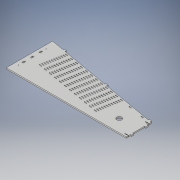
# Autodesk Inventor part: pinball-case-left-wall
Saved by Autodesk Inventor 2017 (Build 210142000, 142)
## iProperties
Created: 2017-02-27
Part Number: pinball-case-left-wall
Material: Generic
Document SubType Name: Modeling
Designer: John
Density: 1 g/cm^3
Appearance: Default
Author: John
Autodesk Inventor part; units mm, degrees
ref_plane "YZ Plane" through (0, 0, 0) normal (1, 0, 0) x (0, 1, 0)
ref_plane "XZ Plane" through (0, 0, 0) normal (0, 1, 0) x (-1, 0, 0)
ref_plane "XY Plane" through (0, 0, 0) normal (0, 0, 1) x (1, 0, 0)
sketch "Sketch1" plane through (0, 0, 0) normal (0, 1, 0) x (-1, 0, 0)
  line L0 (0, 0) -> (-590, 0)
  line L1 (-590, 0) -> (-590, -120.9671)
  line L2 (-590, -120.9671) -> (0, -120.9671)
  line L3 (0, -120.9671) -> (0, 0)
  line L4 (0, -120.9671) -> (0, -225)
  line L5 (0, -225) -> (-590, -120.9671)
  dimension "d0" = 590
  dimension "d50" = 225
  dimension "d51" = 10
  constraints: 12 end point, 2 parallel, 1 horizontal, 1 perpendicular, 1 vertical
  measures "d0" distance of L2.end L1.end
  measures "d50" distance of L0.start L4.end
  measures "d51" angle of L2 L5
extrude "Extrusion1" add sketch "Sketch1" along normal blind 6
sketch "Sketch2" plane through (0, 6, 0) normal (0, 1, 0) x (1, 0, 0)
  line L0 (62.143, 214.0425) -> (73.9607, 211.9587)
  line L1 (73.9607, 211.9587) -> (75.0026, 217.8676)
  line L2 (75.0026, 217.8676) -> (63.1849, 219.9514)
  line L3 (63.1849, 219.9514) -> (62.143, 214.0425)
  line L4 (0, 225) -> (62.143, 214.0425) construction
  line L5 (590, 120.9671) -> (578.1823, 123.0509) construction
  line L6 (590, 120.9671) -> (0, 225) construction
  line L7 (578.1823, 123.0509) -> (566.3646, 125.1346)
  line L8 (566.3646, 125.1346) -> (567.4065, 131.0435)
  line L9 (567.4065, 131.0435) -> (579.2242, 128.9597)
  line L10 (579.2242, 128.9597) -> (578.1823, 123.0509)
  line L11 (320.1627, 168.5467) -> (308.345, 170.6305)
  line L12 (308.345, 170.6305) -> (309.3869, 176.5393)
  line L13 (309.3869, 176.5393) -> (321.2046, 174.4555)
  line L14 (321.2046, 174.4555) -> (320.1627, 168.5467)
  point P0 (0, 0)
  dimension "d5" = 6
  dimension "d7" = 12
  dimension "d9" = 12
  dimension "d10" = 12
  dimension "d11" = 6
  dimension "d14" = 500
  dimension "d15" = 12
  dimension "d16" = 6
  dimension "d17" = 250
  constraints: 28 end point, 6 parallel, 3 perpendicular, 3 point on line, 1 collinear
  measures "d5" distance of L1.end L0.end
  measures "d7" distance between parallel lines of L1 L3
  measures "d9" distance of L5.start L5.end
  measures "d10" distance of L5.end L7.end
  measures "d11" distance of L7.end L8.end
  measures "d14" distance between parallel lines of L8 L1
  measures "d15" distance of L11.start L11.end
  measures "d16" distance of L11.end L12.end
  measures "d17" distance between parallel lines of L14 L8
extrude "Extrusion2" add sketch "Sketch2" against normal blind 6
sketch "Sketch3" plane through (0, 6, 0) normal (0, 1, 0) x (1, 0, 0)
  line L0 (590, 0) -> (590, 120.9671) projected
  line L1 (590, 126) -> (584, 126)
  line L2 (584, 126) -> (584, 101)
  line L3 (584, 101) -> (590, 101)
  line L4 (590, 101) -> (590, 126)
  line L5 (590, 0) -> (584, 0)
  line L6 (584, 0) -> (584, 20)
  line L7 (584, 20) -> (590, 20)
  line L8 (590, 20) -> (590, 0)
  line L9 (590, 89) -> (584, 89)
  line L10 (584, 89) -> (584, 32)
  line L11 (584, 32) -> (590, 32)
  line L12 (590, 32) -> (590, 89)
  point P0 (0, 0)
  dimension "d18" = 6
  dimension "d20" = 6
  dimension "d21" = 20
  dimension "d22" = 12
  dimension "d23" = 12
  dimension "d27" = 57
  dimension "d36" = 25
  constraints: 24 end point, 6 parallel, 3 horizontal, 3 perpendicular, 1 point on line
  measures "d18" distance of L3.end L2.end
  measures "d20" distance of L6.end L7.end
  measures "d21" distance of L5.end L6.end
  measures "d22" distance between parallel lines of L3 L9
  measures "d23" distance between parallel lines of L7 L11
  measures "d27" distance of L9.end L10.end
  measures "d36" distance of L1.end L2.end
extrude "Extrusion3" cut sketch "Sketch3" along normal through all both and the other way through all
sketch "Sketch4" plane through (0, 6, 0) normal (0, 1, 0) x (1, 0, 0)
  line L0 (584, 0) -> (584, 20) projected
  line L1 (584, 12) -> (576, 12)
  line L2 (567, 12) -> (567, 9.5)
  line L3 (567, 9.5) -> (573.7, 9.5)
  line L4 (584, 9.5) -> (584, 12)
  line L5 (0, 0) -> (584, 0) construction
  line L6 (573.7, 13.45) -> (576, 13.45)
  line L7 (576, 13.45) -> (576, 12)
  line L8 (576, 8.05) -> (573.7, 8.05)
  line L9 (573.7, 8.05) -> (573.7, 9.5)
  line L10 (576, 12) -> (576, 9.5) construction
  line L11 (576, 9.5) -> (576, 8.05)
  line L12 (573.7, 12) -> (573.7, 13.45)
  line L13 (573.7, 9.5) -> (573.7, 12) construction
  line L14 (576, 12) -> (573.7, 12) construction
  line L15 (573.7, 12) -> (567, 12)
  line L16 (576, 9.5) -> (584, 9.5)
  line L17 (573.7, 9.5) -> (576, 9.5) construction
  line L18 (584, 111.5) -> (576, 111.5)
  line L19 (567, 111.5) -> (567, 109)
  line L20 (567, 109) -> (573.7, 109)
  line L21 (584, 109) -> (584, 111.5)
  line L22 (573.7, 112.95) -> (576, 112.95)
  line L23 (576, 112.95) -> (576, 111.5)
  line L24 (576, 107.55) -> (573.7, 107.55)
  line L25 (573.7, 107.55) -> (573.7, 109)
  line L26 (576, 111.5) -> (576, 109) construction
  line L27 (576, 109) -> (576, 107.55)
  line L28 (573.7, 111.5) -> (573.7, 112.95)
  line L29 (573.7, 109) -> (573.7, 111.5) construction
  line L30 (576, 111.5) -> (573.7, 111.5) construction
  line L31 (573.7, 111.5) -> (567, 111.5)
  line L32 (576, 109) -> (584, 109)
  line L33 (573.7, 109) -> (576, 109) construction
  line L34 (590, 101) -> (584, 101) construction
  line L35 (584, 20) -> (590, 20) construction
  line L36 (14.1705, 156) -> (20.1705, 156)
  line L37 (20.1705, 156) -> (20.1705, 144)
  line L38 (20.1705, 144) -> (14.1705, 144)
  line L39 (14.1705, 144) -> (14.1705, 156)
  line L40 (15, 114) -> (21, 114)
  line L41 (21, 114) -> (21, 102)
  line L42 (21, 102) -> (15, 102)
  line L43 (15, 102) -> (15, 114)
  line L44 (15, 72) -> (21, 72)
  line L45 (21, 72) -> (21, 60)
  line L46 (21, 60) -> (15, 60)
  line L47 (15, 60) -> (15, 72)
  line L48 (0, 225) -> (0, 0) projected
  circle A0 centre (17.1705, 176) radius 1.25
  circle A1 centre (18, 40) radius 1.25
  line L49 (18, 60) -> (18, 40) construction
  point P0 (584, 122.025)
  dimension "d37" = 17
  dimension "d38" = 2.5
  dimension "d58" = 2.3
  dimension "d59" = 5.4
  dimension "d60" = 8
  dimension "d66" = 17
  dimension "d67" = 2.5
  dimension "d68" = 2.3
  dimension "d69" = 5.4
  dimension "d70" = 8
  dimension "d71" = 8
  dimension "d72" = 6
  dimension "d73" = 12
  dimension "d77" = 30
  dimension "d78" = 30
  dimension "d79" = 60
  dimension "d80" = 15
  dimension "d81" = 2.5
  dimension "d82" = 2.5
  dimension "d83" = 20
  dimension "d84" = 20
  constraints: 90 end point, 46 parallel, 15 perpendicular, 11 horizontal, 5 equal length, 5 point on line, 2 centre point, 1 midpoint, 1 vertical
  measures "d37" distance of L4.start L2.end
  measures "d38" distance of L2.end L2.start
  measures "d58" distance of L8.start L8.end
  measures "d59" distance of L6.end L8.start
  measures "d60" distance between parallel lines of L0 L7
  measures "d66" distance of L21.start L19.end
  measures "d67" distance of L19.end L31.end
  measures "d68" distance of L24.start L24.end
  measures "d69" distance of L22.end L24.start
  measures "d70" distance between parallel lines of L34 L32
  measures "d71" distance between parallel lines of L1 L35
  measures "d72" distance of L37.end L38.end
  measures "d73" distance of L36.end L37.end
  measures "d77" distance between parallel lines of L38 L40
  measures "d78" distance between parallel lines of L44 L42
  measures "d79" distance between parallel lines of L46 L5
  measures "d80" distance between parallel lines of L48 L47
  measures "d81" diameter of A0
  measures "d82" diameter of A1
  measures "d83" distance from line of L49.end L46
  measures "d84" distance from line of L36 A0.centre
extrude "Extrusion4" cut sketch "Sketch4" along normal through all both and the other way through all
sketch "Sketch5" plane through (0, 6, 0) normal (0, 1, 0) x (1, 0, 0)
  circle A0 centre (490, 60) radius 12
  line L0 (0, 0) -> (584, 0) projected
  line L1 (590, 89) -> (590, 101) projected
  dimension "d45" = 24
  dimension "d46" = 60
  dimension "d47" = 100
  constraints: 1 centre point
  measures "d45" diameter of A0
  measures "d46" distance from line of L0 A0.centre
  measures "d47" distance from line of L1 A0.centre
extrude "Extrusion5" cut sketch "Sketch5" against normal through all
sketch "Sketch6" plane through (0, 6, 0) normal (0, 1, 0) x (1, 0, 0)
  line L0 (533.8089, 124.7825) -> (545.6266, 122.6988)
  line L1 (545.6266, 122.6988) -> (545.1056, 119.7443)
  line L2 (545.1056, 119.7443) -> (533.2879, 121.8281)
  line L3 (533.2879, 121.8281) -> (533.8089, 124.7825)
  line L4 (474.7204, 135.2014) -> (462.9027, 137.2852)
  line L5 (462.9027, 137.2852) -> (462.3818, 134.3308)
  line L6 (462.3818, 134.3308) -> (474.1995, 132.247)
  line L7 (474.1995, 132.247) -> (474.7204, 135.2014)
  line L8 (566.3646, 125.1346) -> (320.1627, 168.5467) projected
  point P0 (0, 0)
  dimension "d85" = 12
  dimension "d86" = 3
  dimension "d87" = 12
  dimension "d88" = 60
  dimension "d89" = 20
  dimension "d92" = 6
  constraints: 16 end point, 5 parallel, 2 perpendicular, 2 point on line, 1 collinear
  measures "d85" distance of L1.end L2.end
  measures "d86" distance of L0.end L1.end
  measures "d87" distance of L6.end L5.end
  measures "d88" distance between parallel lines of L7 L3
  measures "d89" distance from line of L1 L8.start
  measures "d92" distance between parallel lines of L0 L8
extrude "Extrusion6" cut sketch "Sketch6" against normal through all
sketch "Sketch7" plane through (0, 6, 0) normal (0, 1, 0) x (1, 0, 0)
  line L0 (422.9895, 141.2767) -> (411.1718, 143.3605)
  line L1 (411.1718, 143.3605) -> (411.6927, 146.3149)
  line L2 (411.6927, 146.3149) -> (423.5104, 144.2311)
  line L3 (423.5104, 144.2311) -> (422.9895, 141.2767)
  line L4 (462.9027, 137.2852) -> (474.7204, 135.2014) projected
  line L5 (566.3646, 125.1346) -> (320.1627, 168.5467) projected
  line L6 (421.253, 131.4286) -> (409.4353, 133.5124)
  line L7 (409.4353, 133.5124) -> (409.9562, 136.4668)
  line L8 (409.9562, 136.4668) -> (421.7739, 134.3831)
  line L9 (421.7739, 134.3831) -> (421.253, 131.4286)
  line L10 (419.5165, 121.5806) -> (407.6988, 123.6643)
  line L11 (407.6988, 123.6643) -> (408.2198, 126.6188)
  line L12 (408.2198, 126.6188) -> (420.0374, 124.535)
  line L13 (420.0374, 124.535) -> (419.5165, 121.5806)
  line L14 (417.78, 111.7325) -> (405.9623, 113.8163)
  line L15 (405.9623, 113.8163) -> (406.4833, 116.7707)
  line L16 (406.4833, 116.7707) -> (418.301, 114.6869)
  line L17 (418.301, 114.6869) -> (417.78, 111.7325)
  line L18 (416.0435, 101.8844) -> (404.2258, 103.9682)
  line L19 (404.2258, 103.9682) -> (404.7468, 106.9226)
  line L20 (404.7468, 106.9226) -> (416.5645, 104.8388)
  line L21 (416.5645, 104.8388) -> (416.0435, 101.8844)
  line L22 (414.3071, 92.0363) -> (402.4894, 94.1201)
  line L23 (402.4894, 94.1201) -> (403.0103, 97.0745)
  line L24 (403.0103, 97.0745) -> (414.828, 94.9907)
  line L25 (414.828, 94.9907) -> (414.3071, 92.0363)
  line L26 (412.5706, 82.1882) -> (400.7529, 84.272)
  line L27 (400.7529, 84.272) -> (401.2738, 87.2264)
  line L28 (401.2738, 87.2264) -> (413.0915, 85.1427)
  line L29 (413.0915, 85.1427) -> (412.5706, 82.1882)
  line L30 (410.8341, 72.3402) -> (399.0164, 74.4239)
  line L31 (399.0164, 74.4239) -> (399.5373, 77.3784)
  line L32 (399.5373, 77.3784) -> (411.355, 75.2946)
  line L33 (411.355, 75.2946) -> (410.8341, 72.3402)
  line L34 (393.4452, 146.4862) -> (381.6275, 148.5699)
  line L35 (381.6275, 148.5699) -> (382.1485, 151.5244)
  line L36 (382.1485, 151.5244) -> (393.9662, 149.4406)
  line L37 (393.9662, 149.4406) -> (393.4452, 146.4862)
  line L38 (391.7087, 136.6381) -> (379.8911, 138.7219)
  line L39 (379.8911, 138.7219) -> (380.412, 141.6763)
  line L40 (380.412, 141.6763) -> (392.2297, 139.5925)
  line L41 (392.2297, 139.5925) -> (391.7087, 136.6381)
  line L42 (389.9723, 126.79) -> (378.1546, 128.8738)
  line L43 (378.1546, 128.8738) -> (378.6755, 131.8282)
  line L44 (378.6755, 131.8282) -> (390.4932, 129.7444)
  line L45 (390.4932, 129.7444) -> (389.9723, 126.79)
  line L46 (388.2358, 116.9419) -> (376.4181, 119.0257)
  line L47 (376.4181, 119.0257) -> (376.939, 121.9801)
  line L48 (376.939, 121.9801) -> (388.7567, 119.8963)
  line L49 (388.7567, 119.8963) -> (388.2358, 116.9419)
  line L50 (386.4993, 107.0938) -> (374.6816, 109.1776)
  line L51 (374.6816, 109.1776) -> (375.2026, 112.132)
  line L52 (375.2026, 112.132) -> (387.0202, 110.0483)
  line L53 (387.0202, 110.0483) -> (386.4993, 107.0938)
  line L54 (384.7628, 97.2458) -> (372.9451, 99.3295)
  line L55 (372.9451, 99.3295) -> (373.4661, 102.284)
  line L56 (373.4661, 102.284) -> (385.2838, 100.2002)
  line L57 (385.2838, 100.2002) -> (384.7628, 97.2458)
  line L58 (383.0263, 87.3977) -> (371.2086, 89.4815)
  line L59 (371.2086, 89.4815) -> (371.7296, 92.4359)
  line L60 (371.7296, 92.4359) -> (383.5473, 90.3521)
  line L61 (383.5473, 90.3521) -> (383.0263, 87.3977)
  line L62 (381.2899, 77.5496) -> (369.4722, 79.6334)
  line L63 (369.4722, 79.6334) -> (369.9931, 82.5878)
  line L64 (369.9931, 82.5878) -> (381.8108, 80.504)
  line L65 (381.8108, 80.504) -> (381.2899, 77.5496)
  line L66 (363.901, 151.6956) -> (352.0833, 153.7794)
  line L67 (352.0833, 153.7794) -> (352.6043, 156.7338)
  line L68 (352.6043, 156.7338) -> (364.4219, 154.65)
  line L69 (364.4219, 154.65) -> (363.901, 151.6956)
  line L70 (362.1645, 141.8475) -> (350.3468, 143.9313)
  line L71 (350.3468, 143.9313) -> (350.8678, 146.8857)
  line L72 (350.8678, 146.8857) -> (362.6855, 144.8019)
  line L73 (362.6855, 144.8019) -> (362.1645, 141.8475)
  line L74 (360.428, 131.9994) -> (348.6103, 134.0832)
  line L75 (348.6103, 134.0832) -> (349.1313, 137.0376)
  line L76 (349.1313, 137.0376) -> (360.949, 134.9539)
  line L77 (360.949, 134.9539) -> (360.428, 131.9994)
  line L78 (358.6916, 122.1514) -> (346.8739, 124.2351)
  line L79 (346.8739, 124.2351) -> (347.3948, 127.1896)
  line L80 (347.3948, 127.1896) -> (359.2125, 125.1058)
  line L81 (359.2125, 125.1058) -> (358.6916, 122.1514)
  line L82 (356.9551, 112.3033) -> (345.1374, 114.3871)
  line L83 (345.1374, 114.3871) -> (345.6583, 117.3415)
  line L84 (345.6583, 117.3415) -> (357.476, 115.2577)
  line L85 (357.476, 115.2577) -> (356.9551, 112.3033)
  line L86 (355.2186, 102.4552) -> (343.4009, 104.539)
  line L87 (343.4009, 104.539) -> (343.9218, 107.4934)
  line L88 (343.9218, 107.4934) -> (355.7395, 105.4096)
  line L89 (355.7395, 105.4096) -> (355.2186, 102.4552)
  line L90 (353.4821, 92.6071) -> (341.6644, 94.6909)
  line L91 (341.6644, 94.6909) -> (342.1854, 97.6453)
  line L92 (342.1854, 97.6453) -> (354.0031, 95.5616)
  line L93 (354.0031, 95.5616) -> (353.4821, 92.6071)
  line L94 (351.7456, 82.7591) -> (339.9279, 84.8428)
  line L95 (339.9279, 84.8428) -> (340.4489, 87.7973)
  line L96 (340.4489, 87.7973) -> (352.2666, 85.7135)
  line L97 (352.2666, 85.7135) -> (351.7456, 82.7591)
  line L98 (334.3568, 156.905) -> (322.5391, 158.9888)
  line L99 (322.5391, 158.9888) -> (323.06, 161.9432)
  line L100 (323.06, 161.9432) -> (334.8777, 159.8595)
  line L101 (334.8777, 159.8595) -> (334.3568, 156.905)
  line L102 (332.6203, 147.057) -> (320.8026, 149.1407)
  line L103 (320.8026, 149.1407) -> (321.3235, 152.0952)
  line L104 (321.3235, 152.0952) -> (333.1412, 150.0114)
  line L105 (333.1412, 150.0114) -> (332.6203, 147.057)
  line L106 (330.8838, 137.2089) -> (319.0661, 139.2927)
  line L107 (319.0661, 139.2927) -> (319.5871, 142.2471)
  line L108 (319.5871, 142.2471) -> (331.4047, 140.1633)
  line L109 (331.4047, 140.1633) -> (330.8838, 137.2089)
  line L110 (329.1473, 127.3608) -> (317.3296, 129.4446)
  line L111 (317.3296, 129.4446) -> (317.8506, 132.399)
  line L112 (317.8506, 132.399) -> (329.6683, 130.3152)
  line L113 (329.6683, 130.3152) -> (329.1473, 127.3608)
  line L114 (327.4108, 117.5127) -> (315.5931, 119.5965)
  line L115 (315.5931, 119.5965) -> (316.1141, 122.5509)
  line L116 (316.1141, 122.5509) -> (327.9318, 120.4672)
  line L117 (327.9318, 120.4672) -> (327.4108, 117.5127)
  line L118 (325.6744, 107.6647) -> (313.8567, 109.7484)
  line L119 (313.8567, 109.7484) -> (314.3776, 112.7029)
  line L120 (314.3776, 112.7029) -> (326.1953, 110.6191)
  line L121 (326.1953, 110.6191) -> (325.6744, 107.6647)
  line L122 (323.9379, 97.8166) -> (312.1202, 99.9004)
  line L123 (312.1202, 99.9004) -> (312.6411, 102.8548)
  line L124 (312.6411, 102.8548) -> (324.4588, 100.771)
  line L125 (324.4588, 100.771) -> (323.9379, 97.8166)
  line L126 (322.2014, 87.9685) -> (310.3837, 90.0523)
  line L127 (310.3837, 90.0523) -> (310.9046, 93.0067)
  line L128 (310.9046, 93.0067) -> (322.7223, 90.9229)
  line L129 (322.7223, 90.9229) -> (322.2014, 87.9685)
  line L130 (304.8125, 162.1145) -> (292.9948, 164.1983)
  line L131 (292.9948, 164.1983) -> (293.5158, 167.1527)
  line L132 (293.5158, 167.1527) -> (305.3335, 165.0689)
  line L133 (305.3335, 165.0689) -> (304.8125, 162.1145)
  line L134 (303.0761, 152.2664) -> (291.2584, 154.3502)
  line L135 (291.2584, 154.3502) -> (291.7793, 157.3046)
  line L136 (291.7793, 157.3046) -> (303.597, 155.2208)
  line L137 (303.597, 155.2208) -> (303.0761, 152.2664)
  line L138 (301.3396, 142.4183) -> (289.5219, 144.5021)
  line L139 (289.5219, 144.5021) -> (290.0428, 147.4565)
  line L140 (290.0428, 147.4565) -> (301.8605, 145.3728)
  line L141 (301.8605, 145.3728) -> (301.3396, 142.4183)
  line L142 (299.6031, 132.5703) -> (287.7854, 134.654)
  line L143 (287.7854, 134.654) -> (288.3063, 137.6085)
  line L144 (288.3063, 137.6085) -> (300.124, 135.5247)
  line L145 (300.124, 135.5247) -> (299.6031, 132.5703)
  line L146 (297.8666, 122.7222) -> (286.0489, 124.806)
  line L147 (286.0489, 124.806) -> (286.5699, 127.7604)
  line L148 (286.5699, 127.7604) -> (298.3876, 125.6766)
  line L149 (298.3876, 125.6766) -> (297.8666, 122.7222)
  line L150 (296.1301, 112.8741) -> (284.3124, 114.9579)
  line L151 (284.3124, 114.9579) -> (284.8334, 117.9123)
  line L152 (284.8334, 117.9123) -> (296.6511, 115.8285)
  line L153 (296.6511, 115.8285) -> (296.1301, 112.8741)
  line L154 (294.3936, 103.026) -> (282.5759, 105.1098)
  line L155 (282.5759, 105.1098) -> (283.0969, 108.0642)
  line L156 (283.0969, 108.0642) -> (294.9146, 105.9804)
  line L157 (294.9146, 105.9804) -> (294.3936, 103.026)
  line L158 (292.6572, 93.1779) -> (280.8395, 95.2617)
  line L159 (280.8395, 95.2617) -> (281.3604, 98.2161)
  line L160 (281.3604, 98.2161) -> (293.1781, 96.1324)
  line L161 (293.1781, 96.1324) -> (292.6572, 93.1779)
  line L162 (275.2683, 167.3239) -> (263.4506, 169.4077)
  line L163 (263.4506, 169.4077) -> (263.9716, 172.3621)
  line L164 (263.9716, 172.3621) -> (275.7892, 170.2784)
  line L165 (275.7892, 170.2784) -> (275.2683, 167.3239)
  line L166 (273.5318, 157.4759) -> (261.7141, 159.5596)
  line L167 (261.7141, 159.5596) -> (262.2351, 162.5141)
  line L168 (262.2351, 162.5141) -> (274.0528, 160.4303)
  line L169 (274.0528, 160.4303) -> (273.5318, 157.4759)
  line L170 (271.7953, 147.6278) -> (259.9776, 149.7116)
  line L171 (259.9776, 149.7116) -> (260.4986, 152.666)
  line L172 (260.4986, 152.666) -> (272.3163, 150.5822)
  line L173 (272.3163, 150.5822) -> (271.7953, 147.6278)
  line L174 (270.0589, 137.7797) -> (258.2412, 139.8635)
  line L175 (258.2412, 139.8635) -> (258.7621, 142.8179)
  line L176 (258.7621, 142.8179) -> (270.5798, 140.7341)
  line L177 (270.5798, 140.7341) -> (270.0589, 137.7797)
  line L178 (268.3224, 127.9316) -> (256.5047, 130.0154)
  line L179 (256.5047, 130.0154) -> (257.0256, 132.9698)
  line L180 (257.0256, 132.9698) -> (268.8433, 130.886)
  line L181 (268.8433, 130.886) -> (268.3224, 127.9316)
  line L182 (266.5859, 118.0835) -> (254.7682, 120.1673)
  line L183 (254.7682, 120.1673) -> (255.2891, 123.1217)
  line L184 (255.2891, 123.1217) -> (267.1068, 121.038)
  line L185 (267.1068, 121.038) -> (266.5859, 118.0835)
  line L186 (264.8494, 108.2355) -> (253.0317, 110.3192)
  line L187 (253.0317, 110.3192) -> (253.5527, 113.2737)
  line L188 (253.5527, 113.2737) -> (265.3704, 111.1899)
  line L189 (265.3704, 111.1899) -> (264.8494, 108.2355)
  line L190 (263.1129, 98.3874) -> (251.2952, 100.4712)
  line L191 (251.2952, 100.4712) -> (251.8162, 103.4256)
  line L192 (251.8162, 103.4256) -> (263.6339, 101.3418)
  line L193 (263.6339, 101.3418) -> (263.1129, 98.3874)
  line L194 (245.7241, 172.5334) -> (233.9064, 174.6172)
  line L195 (233.9064, 174.6172) -> (234.4273, 177.5716)
  line L196 (234.4273, 177.5716) -> (246.245, 175.4878)
  line L197 (246.245, 175.4878) -> (245.7241, 172.5334)
  line L198 (243.9876, 162.6853) -> (232.1699, 164.7691)
  line L199 (232.1699, 164.7691) -> (232.6908, 167.7235)
  line L200 (232.6908, 167.7235) -> (244.5085, 165.6397)
  line L201 (244.5085, 165.6397) -> (243.9876, 162.6853)
  line L202 (242.2511, 152.8372) -> (230.4334, 154.921)
  line L203 (230.4334, 154.921) -> (230.9544, 157.8754)
  line L204 (230.9544, 157.8754) -> (242.772, 155.7916)
  line L205 (242.772, 155.7916) -> (242.2511, 152.8372)
  line L206 (240.5146, 142.9891) -> (228.6969, 145.0729)
  line L207 (228.6969, 145.0729) -> (229.2179, 148.0273)
  line L208 (229.2179, 148.0273) -> (241.0356, 145.9436)
  line L209 (241.0356, 145.9436) -> (240.5146, 142.9891)
  line L210 (238.7781, 133.1411) -> (226.9604, 135.2248)
  line L211 (226.9604, 135.2248) -> (227.4814, 138.1793)
  line L212 (227.4814, 138.1793) -> (239.2991, 136.0955)
  line L213 (239.2991, 136.0955) -> (238.7781, 133.1411)
  line L214 (237.0417, 123.293) -> (225.224, 125.3768)
  line L215 (225.224, 125.3768) -> (225.7449, 128.3312)
  line L216 (225.7449, 128.3312) -> (237.5626, 126.2474)
  line L217 (237.5626, 126.2474) -> (237.0417, 123.293)
  line L218 (235.3052, 113.4449) -> (223.4875, 115.5287)
  line L219 (223.4875, 115.5287) -> (224.0084, 118.4831)
  line L220 (224.0084, 118.4831) -> (235.8261, 116.3993)
  line L221 (235.8261, 116.3993) -> (235.3052, 113.4449)
  line L222 (233.5687, 103.5968) -> (221.751, 105.6806)
  line L223 (221.751, 105.6806) -> (222.2719, 108.635)
  line L224 (222.2719, 108.635) -> (234.0896, 106.5513)
  line L225 (234.0896, 106.5513) -> (233.5687, 103.5968)
  line L226 (216.1798, 177.7428) -> (204.3621, 179.8266)
  line L227 (204.3621, 179.8266) -> (204.8831, 182.781)
  line L228 (204.8831, 182.781) -> (216.7008, 180.6972)
  line L229 (216.7008, 180.6972) -> (216.1798, 177.7428)
  line L230 (214.4434, 167.8947) -> (202.6257, 169.9785)
  line L231 (202.6257, 169.9785) -> (203.1466, 172.9329)
  line L232 (203.1466, 172.9329) -> (214.9643, 170.8492)
  line L233 (214.9643, 170.8492) -> (214.4434, 167.8947)
  line L234 (212.7069, 158.0467) -> (200.8892, 160.1304)
  line L235 (200.8892, 160.1304) -> (201.4101, 163.0849)
  line L236 (201.4101, 163.0849) -> (213.2278, 161.0011)
  line L237 (213.2278, 161.0011) -> (212.7069, 158.0467)
  line L238 (210.9704, 148.1986) -> (199.1527, 150.2824)
  line L239 (199.1527, 150.2824) -> (199.6736, 153.2368)
  line L240 (199.6736, 153.2368) -> (211.4913, 151.153)
  line L241 (211.4913, 151.153) -> (210.9704, 148.1986)
  line L242 (209.2339, 138.3505) -> (197.4162, 140.4343)
  line L243 (197.4162, 140.4343) -> (197.9372, 143.3887)
  line L244 (197.9372, 143.3887) -> (209.7549, 141.3049)
  line L245 (209.7549, 141.3049) -> (209.2339, 138.3505)
  line L246 (207.4974, 128.5024) -> (195.6797, 130.5862)
  line L247 (195.6797, 130.5862) -> (196.2007, 133.5406)
  line L248 (196.2007, 133.5406) -> (208.0184, 131.4569)
  line L249 (208.0184, 131.4569) -> (207.4974, 128.5024)
  line L250 (205.7609, 118.6544) -> (193.9433, 120.7381)
  line L251 (193.9433, 120.7381) -> (194.4642, 123.6926)
  line L252 (194.4642, 123.6926) -> (206.2819, 121.6088)
  line L253 (206.2819, 121.6088) -> (205.7609, 118.6544)
  line L254 (204.0245, 108.8063) -> (192.2068, 110.8901)
  line L255 (192.2068, 110.8901) -> (192.7277, 113.8445)
  line L256 (192.7277, 113.8445) -> (204.5454, 111.7607)
  line L257 (204.5454, 111.7607) -> (204.0245, 108.8063)
  line L258 (462.3818, 134.3308) -> (462.9027, 137.2852) projected
  line L259 (409.0976, 62.4921) -> (397.2799, 64.5759)
  line L260 (397.2799, 64.5759) -> (397.8009, 67.5303)
  line L261 (397.8009, 67.5303) -> (409.6186, 65.4465)
  line L262 (409.6186, 65.4465) -> (409.0976, 62.4921)
  line L263 (379.5534, 67.7015) -> (367.7357, 69.7853)
  line L264 (367.7357, 69.7853) -> (368.2566, 72.7397)
  line L265 (368.2566, 72.7397) -> (380.0743, 70.656)
  line L266 (380.0743, 70.656) -> (379.5534, 67.7015)
  line L267 (350.0091, 72.911) -> (338.1915, 74.9948)
  line L268 (338.1915, 74.9948) -> (338.7124, 77.9492)
  line L269 (338.7124, 77.9492) -> (350.5301, 75.8654)
  line L270 (350.5301, 75.8654) -> (350.0091, 72.911)
  line L271 (320.4649, 78.1204) -> (308.6472, 80.2042)
  line L272 (308.6472, 80.2042) -> (309.1682, 83.1586)
  line L273 (309.1682, 83.1586) -> (320.9859, 81.0748)
  line L274 (320.9859, 81.0748) -> (320.4649, 78.1204)
  line L275 (290.9207, 83.3299) -> (279.103, 85.4136)
  line L276 (279.103, 85.4136) -> (279.6239, 88.3681)
  line L277 (279.6239, 88.3681) -> (291.4416, 86.2843)
  line L278 (291.4416, 86.2843) -> (290.9207, 83.3299)
  line L279 (261.3764, 88.5393) -> (249.5588, 90.6231)
  line L280 (249.5588, 90.6231) -> (250.0797, 93.5775)
  line L281 (250.0797, 93.5775) -> (261.8974, 91.4937)
  line L282 (261.8974, 91.4937) -> (261.3764, 88.5393)
  line L283 (231.8322, 93.7488) -> (220.0145, 95.8325)
  line L284 (220.0145, 95.8325) -> (220.5355, 98.787)
  line L285 (220.5355, 98.787) -> (232.3532, 96.7032)
  line L286 (232.3532, 96.7032) -> (231.8322, 93.7488)
  line L287 (202.288, 98.9582) -> (190.4703, 101.042)
  line L288 (190.4703, 101.042) -> (190.9912, 103.9964)
  line L289 (190.9912, 103.9964) -> (202.8089, 101.9126)
  line L290 (202.8089, 101.9126) -> (202.288, 98.9582)
  line L291 (407.3611, 52.644) -> (395.5434, 54.7278)
  line L292 (395.5434, 54.7278) -> (396.0644, 57.6822)
  line L293 (396.0644, 57.6822) -> (407.8821, 55.5984)
  line L294 (407.8821, 55.5984) -> (407.3611, 52.644)
  line L295 (377.8169, 57.8535) -> (365.9992, 59.9372)
  line L296 (365.9992, 59.9372) -> (366.5201, 62.8917)
  line L297 (366.5201, 62.8917) -> (378.3378, 60.8079)
  line L298 (378.3378, 60.8079) -> (377.8169, 57.8535)
  line L299 (348.2727, 63.0629) -> (336.455, 65.1467)
  line L300 (336.455, 65.1467) -> (336.9759, 68.1011)
  line L301 (336.9759, 68.1011) -> (348.7936, 66.0173)
  line L302 (348.7936, 66.0173) -> (348.2727, 63.0629)
  line L303 (318.7284, 68.2723) -> (306.9107, 70.3561)
  line L304 (306.9107, 70.3561) -> (307.4317, 73.3105)
  line L305 (307.4317, 73.3105) -> (319.2494, 71.2268)
  line L306 (319.2494, 71.2268) -> (318.7284, 68.2723)
  line L307 (289.1842, 73.4818) -> (277.3665, 75.5656)
  line L308 (277.3665, 75.5656) -> (277.8874, 78.52)
  line L309 (277.8874, 78.52) -> (289.7051, 76.4362)
  line L310 (289.7051, 76.4362) -> (289.1842, 73.4818)
  line L311 (259.64, 78.6912) -> (247.8223, 80.775)
  line L312 (247.8223, 80.775) -> (248.3432, 83.7294)
  line L313 (248.3432, 83.7294) -> (260.1609, 81.6457)
  line L314 (260.1609, 81.6457) -> (259.64, 78.6912)
  line L315 (230.0957, 83.9007) -> (218.278, 85.9845)
  line L316 (218.278, 85.9845) -> (218.799, 88.9389)
  line L317 (218.799, 88.9389) -> (230.6167, 86.8551)
  line L318 (230.6167, 86.8551) -> (230.0957, 83.9007)
  line L319 (200.5515, 89.1101) -> (188.7338, 91.1939)
  line L320 (188.7338, 91.1939) -> (189.2548, 94.1483)
  line L321 (189.2548, 94.1483) -> (201.0724, 92.0645)
  line L322 (201.0724, 92.0645) -> (200.5515, 89.1101)
  line L323 (405.6246, 42.7959) -> (393.807, 44.8797)
  line L324 (393.807, 44.8797) -> (394.3279, 47.8341)
  line L325 (394.3279, 47.8341) -> (406.1456, 45.7504)
  line L326 (406.1456, 45.7504) -> (405.6246, 42.7959)
  line L327 (376.0804, 48.0054) -> (364.2627, 50.0892)
  line L328 (364.2627, 50.0892) -> (364.7837, 53.0436)
  line L329 (364.7837, 53.0436) -> (376.6014, 50.9598)
  line L330 (376.6014, 50.9598) -> (376.0804, 48.0054)
  line L331 (346.5362, 53.2148) -> (334.7185, 55.2986)
  line L332 (334.7185, 55.2986) -> (335.2394, 58.253)
  line L333 (335.2394, 58.253) -> (347.0571, 56.1692)
  line L334 (347.0571, 56.1692) -> (346.5362, 53.2148)
  line L335 (316.9919, 58.4243) -> (305.1743, 60.508)
  line L336 (305.1743, 60.508) -> (305.6952, 63.4625)
  line L337 (305.6952, 63.4625) -> (317.5129, 61.3787)
  line L338 (317.5129, 61.3787) -> (316.9919, 58.4243)
  line L339 (287.4477, 63.6337) -> (275.63, 65.7175)
  line L340 (275.63, 65.7175) -> (276.151, 68.6719)
  line L341 (276.151, 68.6719) -> (287.9687, 66.5881)
  line L342 (287.9687, 66.5881) -> (287.4477, 63.6337)
  line L343 (257.9035, 68.8432) -> (246.0858, 70.9269)
  line L344 (246.0858, 70.9269) -> (246.6067, 73.8814)
  line L345 (246.6067, 73.8814) -> (258.4244, 71.7976)
  line L346 (258.4244, 71.7976) -> (257.9035, 68.8432)
  line L347 (228.3593, 74.0526) -> (216.5416, 76.1364)
  line L348 (216.5416, 76.1364) -> (217.0625, 79.0908)
  line L349 (217.0625, 79.0908) -> (228.8802, 77.007)
  line L350 (228.8802, 77.007) -> (228.3593, 74.0526)
  line L351 (198.815, 79.262) -> (186.9973, 81.3458)
  line L352 (186.9973, 81.3458) -> (187.5183, 84.3002)
  line L353 (187.5183, 84.3002) -> (199.336, 82.2165)
  line L354 (199.336, 82.2165) -> (198.815, 79.262)
  line L355 (403.8882, 32.9479) -> (392.0705, 35.0316)
  line L356 (392.0705, 35.0316) -> (392.5914, 37.9861)
  line L357 (392.5914, 37.9861) -> (404.4091, 35.9023)
  line L358 (404.4091, 35.9023) -> (403.8882, 32.9479)
  line L359 (374.3439, 38.1573) -> (362.5262, 40.2411)
  line L360 (362.5262, 40.2411) -> (363.0472, 43.1955)
  line L361 (363.0472, 43.1955) -> (374.8649, 41.1117)
  line L362 (374.8649, 41.1117) -> (374.3439, 38.1573)
  line L363 (344.7997, 43.3667) -> (332.982, 45.4505)
  line L364 (332.982, 45.4505) -> (333.503, 48.4049)
  line L365 (333.503, 48.4049) -> (345.3206, 46.3212)
  line L366 (345.3206, 46.3212) -> (344.7997, 43.3667)
  line L367 (315.2555, 48.5762) -> (303.4378, 50.66)
  line L368 (303.4378, 50.66) -> (303.9587, 53.6144)
  line L369 (303.9587, 53.6144) -> (315.7764, 51.5306)
  line L370 (315.7764, 51.5306) -> (315.2555, 48.5762)
  line L371 (285.7112, 53.7856) -> (273.8935, 55.8694)
  line L372 (273.8935, 55.8694) -> (274.4145, 58.8238)
  line L373 (274.4145, 58.8238) -> (286.2322, 56.7401)
  line L374 (286.2322, 56.7401) -> (285.7112, 53.7856)
  line L375 (256.167, 58.9951) -> (244.3493, 61.0789)
  line L376 (244.3493, 61.0789) -> (244.8703, 64.0333)
  line L377 (244.8703, 64.0333) -> (256.6879, 61.9495)
  line L378 (256.6879, 61.9495) -> (256.167, 58.9951)
  line L379 (226.6228, 64.2045) -> (214.8051, 66.2883)
  line L380 (214.8051, 66.2883) -> (215.326, 69.2427)
  line L381 (215.326, 69.2427) -> (227.1437, 67.1589)
  line L382 (227.1437, 67.1589) -> (226.6228, 64.2045)
  line L383 (197.0785, 69.414) -> (185.2608, 71.4977)
  line L384 (185.2608, 71.4977) -> (185.7818, 74.4522)
  line L385 (185.7818, 74.4522) -> (197.5995, 72.3684)
  line L386 (197.5995, 72.3684) -> (197.0785, 69.414)
  line L387 (186.6356, 182.9523) -> (174.8179, 185.036)
  line L388 (174.8179, 185.036) -> (175.3389, 187.9905)
  line L389 (175.3389, 187.9905) -> (187.1565, 185.9067)
  line L390 (187.1565, 185.9067) -> (186.6356, 182.9523)
  line L391 (184.8991, 173.1042) -> (173.0814, 175.188)
  line L392 (173.0814, 175.188) -> (173.6024, 178.1424)
  line L393 (173.6024, 178.1424) -> (185.4201, 176.0586)
  line L394 (185.4201, 176.0586) -> (184.8991, 173.1042)
  line L395 (183.1626, 163.2561) -> (171.3449, 165.3399)
  line L396 (171.3449, 165.3399) -> (171.8659, 168.2943)
  line L397 (171.8659, 168.2943) -> (183.6836, 166.2105)
  line L398 (183.6836, 166.2105) -> (183.1626, 163.2561)
  line L399 (181.4262, 153.408) -> (169.6085, 155.4918)
  line L400 (169.6085, 155.4918) -> (170.1294, 158.4462)
  line L401 (170.1294, 158.4462) -> (181.9471, 156.3625)
  line L402 (181.9471, 156.3625) -> (181.4262, 153.408)
  line L403 (179.6897, 143.56) -> (167.872, 145.6437)
  line L404 (167.872, 145.6437) -> (168.3929, 148.5982)
  line L405 (168.3929, 148.5982) -> (180.2106, 146.5144)
  line L406 (180.2106, 146.5144) -> (179.6897, 143.56)
  line L407 (177.9532, 133.7119) -> (166.1355, 135.7957)
  line L408 (166.1355, 135.7957) -> (166.6564, 138.7501)
  line L409 (166.6564, 138.7501) -> (178.4741, 136.6663)
  line L410 (178.4741, 136.6663) -> (177.9532, 133.7119)
  line L411 (176.2167, 123.8638) -> (164.399, 125.9476)
  line L412 (164.399, 125.9476) -> (164.92, 128.902)
  line L413 (164.92, 128.902) -> (176.7377, 126.8182)
  line L414 (176.7377, 126.8182) -> (176.2167, 123.8638)
  line L415 (174.4802, 114.0157) -> (162.6625, 116.0995)
  line L416 (162.6625, 116.0995) -> (163.1835, 119.0539)
  line L417 (163.1835, 119.0539) -> (175.0012, 116.9701)
  line L418 (175.0012, 116.9701) -> (174.4802, 114.0157)
  line L419 (172.7437, 104.1676) -> (160.9261, 106.2514)
  line L420 (160.9261, 106.2514) -> (161.447, 109.2058)
  line L421 (161.447, 109.2058) -> (173.2647, 107.1221)
  line L422 (173.2647, 107.1221) -> (172.7437, 104.1676)
  line L423 (171.0073, 94.3196) -> (159.1896, 96.4033)
  line L424 (159.1896, 96.4033) -> (159.7105, 99.3578)
  line L425 (159.7105, 99.3578) -> (171.5282, 97.274)
  line L426 (171.5282, 97.274) -> (171.0073, 94.3196)
  line L427 (169.2708, 84.4715) -> (157.4531, 86.5553)
  line L428 (157.4531, 86.5553) -> (157.974, 89.5097)
  line L429 (157.974, 89.5097) -> (169.7917, 87.4259)
  line L430 (169.7917, 87.4259) -> (169.2708, 84.4715)
  line L431 (167.5343, 74.6234) -> (155.7166, 76.7072)
  line L432 (155.7166, 76.7072) -> (156.2376, 79.6616)
  line L433 (156.2376, 79.6616) -> (168.0552, 77.5778)
  line L434 (168.0552, 77.5778) -> (167.5343, 74.6234)
  line L435 (157.0914, 188.1617) -> (145.2737, 190.2455)
  line L436 (145.2737, 190.2455) -> (145.7946, 193.1999)
  line L437 (145.7946, 193.1999) -> (157.6123, 191.1161)
  line L438 (157.6123, 191.1161) -> (157.0914, 188.1617)
  line L439 (155.3549, 178.3136) -> (143.5372, 180.3974)
  line L440 (143.5372, 180.3974) -> (144.0581, 183.3518)
  line L441 (144.0581, 183.3518) -> (155.8758, 181.2681)
  line L442 (155.8758, 181.2681) -> (155.3549, 178.3136)
  line L443 (153.6184, 168.4656) -> (141.8007, 170.5493)
  line L444 (141.8007, 170.5493) -> (142.3217, 173.5038)
  line L445 (142.3217, 173.5038) -> (154.1394, 171.42)
  line L446 (154.1394, 171.42) -> (153.6184, 168.4656)
  line L447 (151.8819, 158.6175) -> (140.0642, 160.7013)
  line L448 (140.0642, 160.7013) -> (140.5852, 163.6557)
  line L449 (140.5852, 163.6557) -> (152.4029, 161.5719)
  line L450 (152.4029, 161.5719) -> (151.8819, 158.6175)
  line L451 (150.1454, 148.7694) -> (138.3278, 150.8532)
  line L452 (138.3278, 150.8532) -> (138.8487, 153.8076)
  line L453 (138.8487, 153.8076) -> (150.6664, 151.7238)
  line L454 (150.6664, 151.7238) -> (150.1454, 148.7694)
  line L455 (148.409, 138.9213) -> (136.5913, 141.0051)
  line L456 (136.5913, 141.0051) -> (137.1122, 143.9595)
  line L457 (137.1122, 143.9595) -> (148.9299, 141.8757)
  line L458 (148.9299, 141.8757) -> (148.409, 138.9213)
  line L459 (146.6725, 129.0732) -> (134.8548, 131.157)
  line L460 (134.8548, 131.157) -> (135.3757, 134.1114)
  line L461 (135.3757, 134.1114) -> (147.1934, 132.0277)
  line L462 (147.1934, 132.0277) -> (146.6725, 129.0732)
  line L463 (144.936, 119.2252) -> (133.1183, 121.3089)
  line L464 (133.1183, 121.3089) -> (133.6392, 124.2634)
  line L465 (133.6392, 124.2634) -> (145.4569, 122.1796)
  line L466 (145.4569, 122.1796) -> (144.936, 119.2252)
  line L467 (143.1995, 109.3771) -> (131.3818, 111.4609)
  line L468 (131.3818, 111.4609) -> (131.9028, 114.4153)
  line L469 (131.9028, 114.4153) -> (143.7205, 112.3315)
  line L470 (143.7205, 112.3315) -> (143.1995, 109.3771)
  line L471 (141.463, 99.529) -> (129.6453, 101.6128)
  line L472 (129.6453, 101.6128) -> (130.1663, 104.5672)
  line L473 (130.1663, 104.5672) -> (141.984, 102.4834)
  line L474 (141.984, 102.4834) -> (141.463, 99.529)
  line L475 (139.7266, 89.6809) -> (127.9089, 91.7647)
  line L476 (127.9089, 91.7647) -> (128.4298, 94.7191)
  line L477 (128.4298, 94.7191) -> (140.2475, 92.6354)
  line L478 (140.2475, 92.6354) -> (139.7266, 89.6809)
  line L479 (137.9901, 79.8329) -> (126.1724, 81.9166)
  line L480 (126.1724, 81.9166) -> (126.6933, 84.8711)
  line L481 (126.6933, 84.8711) -> (138.511, 82.7873)
  line L482 (138.511, 82.7873) -> (137.9901, 79.8329)
  line L483 (127.5471, 193.3712) -> (115.7294, 195.4549)
  line L484 (115.7294, 195.4549) -> (116.2504, 198.4094)
  line L485 (116.2504, 198.4094) -> (128.0681, 196.3256)
  line L486 (128.0681, 196.3256) -> (127.5471, 193.3712)
  line L487 (125.8107, 183.5231) -> (113.993, 185.6069)
  line L488 (113.993, 185.6069) -> (114.5139, 188.5613)
  line L489 (114.5139, 188.5613) -> (126.3316, 186.4775)
  line L490 (126.3316, 186.4775) -> (125.8107, 183.5231)
  line L491 (124.0742, 173.675) -> (112.2565, 175.7588)
  line L492 (112.2565, 175.7588) -> (112.7774, 178.7132)
  line L493 (112.7774, 178.7132) -> (124.5951, 176.6294)
  line L494 (124.5951, 176.6294) -> (124.0742, 173.675)
  line L495 (122.3377, 163.8269) -> (110.52, 165.9107)
  line L496 (110.52, 165.9107) -> (111.0409, 168.8651)
  line L497 (111.0409, 168.8651) -> (122.8586, 166.7813)
  line L498 (122.8586, 166.7813) -> (122.3377, 163.8269)
  line L499 (120.6012, 153.9788) -> (108.7835, 156.0626)
  line L500 (108.7835, 156.0626) -> (109.3045, 159.0171)
  line L501 (109.3045, 159.0171) -> (121.1222, 156.9333)
  line L502 (121.1222, 156.9333) -> (120.6012, 153.9788)
  line L503 (118.8647, 144.1308) -> (107.047, 146.2145)
  line L504 (107.047, 146.2145) -> (107.568, 149.169)
  line L505 (107.568, 149.169) -> (119.3857, 147.0852)
  line L506 (119.3857, 147.0852) -> (118.8647, 144.1308)
  line L507 (117.1282, 134.2827) -> (105.3106, 136.3665)
  line L508 (105.3106, 136.3665) -> (105.8315, 139.3209)
  line L509 (105.8315, 139.3209) -> (117.6492, 137.2371)
  line L510 (117.6492, 137.2371) -> (117.1282, 134.2827)
  line L511 (115.3918, 124.4346) -> (103.5741, 126.5184)
  line L512 (103.5741, 126.5184) -> (104.095, 129.4728)
  line L513 (104.095, 129.4728) -> (115.9127, 127.389)
  line L514 (115.9127, 127.389) -> (115.3918, 124.4346)
  line L515 (113.6553, 114.5865) -> (101.8376, 116.6703)
  line L516 (101.8376, 116.6703) -> (102.3585, 119.6247)
  line L517 (102.3585, 119.6247) -> (114.1762, 117.541)
  line L518 (114.1762, 117.541) -> (113.6553, 114.5865)
  line L519 (111.9188, 104.7385) -> (100.1011, 106.8222)
  line L520 (100.1011, 106.8222) -> (100.6221, 109.7767)
  line L521 (100.6221, 109.7767) -> (112.4397, 107.6929)
  line L522 (112.4397, 107.6929) -> (111.9188, 104.7385)
  line L523 (110.1823, 94.8904) -> (98.3646, 96.9742)
  line L524 (98.3646, 96.9742) -> (98.8856, 99.9286)
  line L525 (98.8856, 99.9286) -> (110.7033, 97.8448)
  line L526 (110.7033, 97.8448) -> (110.1823, 94.8904)
  line L527 (108.4458, 85.0423) -> (96.6281, 87.1261)
  line L528 (96.6281, 87.1261) -> (97.1491, 90.0805)
  line L529 (97.1491, 90.0805) -> (108.9668, 87.9967)
  line L530 (108.9668, 87.9967) -> (108.4458, 85.0423)
  line L531 (98.0029, 198.5806) -> (86.1852, 200.6644)
  line L532 (86.1852, 200.6644) -> (86.7062, 203.6188)
  line L533 (86.7062, 203.6188) -> (98.5238, 201.535)
  line L534 (98.5238, 201.535) -> (98.0029, 198.5806)
  line L535 (96.2664, 188.7325) -> (84.4487, 190.8163)
  line L536 (84.4487, 190.8163) -> (84.9697, 193.7707)
  line L537 (84.9697, 193.7707) -> (96.7874, 191.6869)
  line L538 (96.7874, 191.6869) -> (96.2664, 188.7325)
  line L539 (94.5299, 178.8844) -> (82.7122, 180.9682)
  line L540 (82.7122, 180.9682) -> (83.2332, 183.9227)
  line L541 (83.2332, 183.9227) -> (95.0509, 181.8389)
  line L542 (95.0509, 181.8389) -> (94.5299, 178.8844)
  line L543 (92.7935, 169.0364) -> (80.9758, 171.1201)
  line L544 (80.9758, 171.1201) -> (81.4967, 174.0746)
  line L545 (81.4967, 174.0746) -> (93.3144, 171.9908)
  line L546 (93.3144, 171.9908) -> (92.7935, 169.0364)
  line L547 (91.057, 159.1883) -> (79.2393, 161.2721)
  line L548 (79.2393, 161.2721) -> (79.7602, 164.2265)
  line L549 (79.7602, 164.2265) -> (91.5779, 162.1427)
  line L550 (91.5779, 162.1427) -> (91.057, 159.1883)
  line L551 (89.3205, 149.3402) -> (77.5028, 151.424)
  line L552 (77.5028, 151.424) -> (78.0237, 154.3784)
  line L553 (78.0237, 154.3784) -> (89.8414, 152.2946)
  line L554 (89.8414, 152.2946) -> (89.3205, 149.3402)
  line L555 (87.584, 139.4921) -> (75.7663, 141.5759)
  line L556 (75.7663, 141.5759) -> (76.2873, 144.5303)
  line L557 (76.2873, 144.5303) -> (88.105, 142.4466)
  line L558 (88.105, 142.4466) -> (87.584, 139.4921)
  line L559 (85.8475, 129.6441) -> (74.0298, 131.7278)
  line L560 (74.0298, 131.7278) -> (74.5508, 134.6823)
  line L561 (74.5508, 134.6823) -> (86.3685, 132.5985)
  line L562 (86.3685, 132.5985) -> (85.8475, 129.6441)
  line L563 (84.1111, 119.796) -> (72.2934, 121.8798)
  line L564 (72.2934, 121.8798) -> (72.8143, 124.8342)
  line L565 (72.8143, 124.8342) -> (84.632, 122.7504)
  line L566 (84.632, 122.7504) -> (84.1111, 119.796)
  line L567 (82.3746, 109.9479) -> (70.5569, 112.0317)
  line L568 (70.5569, 112.0317) -> (71.0778, 114.9861)
  line L569 (71.0778, 114.9861) -> (82.8955, 112.9023)
  line L570 (82.8955, 112.9023) -> (82.3746, 109.9479)
  line L571 (80.6381, 100.0998) -> (68.8204, 102.1836)
  line L572 (68.8204, 102.1836) -> (69.3413, 105.138)
  line L573 (69.3413, 105.138) -> (81.159, 103.0543)
  line L574 (81.159, 103.0543) -> (80.6381, 100.0998)
  line L575 (78.9016, 90.2518) -> (67.0839, 92.3355)
  line L576 (67.0839, 92.3355) -> (67.6049, 95.29)
  line L577 (67.6049, 95.29) -> (79.4226, 93.2062)
  line L578 (79.4226, 93.2062) -> (78.9016, 90.2518)
  point P0 (0, 0)
  dimension "d93" = 12
  dimension "d94" = 3
  dimension "d95" = 6
  dimension "d98" = 10
  dimension "d101" = 30
  dimension "d104" = 40
  constraints: 1152 end point, 3 equal length, 2 collinear, 1 perpendicular, 1144 other
  measures "d93" distance of L1.end L2.end
  measures "d94" distance of L0.end L1.end
  measures "d95" distance between parallel lines of L5 L2
  measures "d98" distance of L0.start L6.start
  measures "d101" distance of L0.start L34.start
  measures "d104" distance between parallel lines of L258 L3
extrude "Extrusion7" cut sketch "Sketch7" along normal through all both and the other way through all
equation "\"d18\" = d20"
equation "\"d23\" = d22"
equation "\"d78\" = d77"
equation "\"d81\" = d82"
equation "\"d84\" = d83"
body "Solid1"
